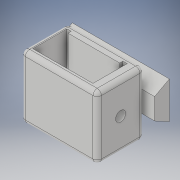
# Autodesk Inventor part: 7.2 Schienenläufer
Saved by Autodesk Inventor 2018.3 (Build 223284000, 284)
## iProperties
Created: 2018-10-11
Part Number: 7.2 Schienenläufer
Material: Generisch
Document SubType Name: Modeling
Designer: pgmadmin
Density: 1 g/cm^3
Appearance: Vorgabe
Author: pgmadmin
Autodesk Inventor part; units mm, degrees
ref_plane "YZ Plane" through (0, 0, 0) normal (1, 0, 0) x (0, 1, 0)
ref_plane "XZ Plane" through (0, 0, 0) normal (0, 1, 0) x (-1, 0, 0)
ref_plane "XY Plane" through (0, 0, 0) normal (0, 0, 1) x (1, 0, 0)
sketch "Skizze1" plane through (0, 0, 0) normal (0, 0, 1) x (1, 0, 0)
  line L0 (-14.1284, 0) -> (-14.1284, 16.2)
  line L1 (-14.1284, 16.2) -> (-12.1284, 16.2)
  line L2 (-12.1284, 16.2) -> (-12.1284, 1.6)
  line L3 (-12.1284, 1.6) -> (12.3716, 1.6)
  line L4 (12.3716, 1.6) -> (12.3716, 16.2)
  line L5 (12.3716, 16.2) -> (14.3716, 16.2)
  line L6 (14.3716, 16.2) -> (14.3716, 0)
  line L7 (14.3716, 0) -> (-14.1284, 0)
  line L8 (-16.6284, 19.2) -> (19.3716, 19.2)
  line L9 (19.3716, 19.2) -> (19.3716, -3)
  line L10 (19.3716, -3) -> (-16.6284, -3)
  line L11 (-16.6284, -3) -> (-16.6284, 19.2)
  line L12 (-12.1284, 14.7) -> (12.3716, 14.7)
  point P0 (0, 0)
  dimension "d1" = 2
  dimension "d3" = 2
  dimension "d4" = 1.6
  dimension "d5" = 3
  dimension "d7" = 2.5
  dimension "d8" = 5
  dimension "d9" = 1.5
  dimension "d26" = 3
  dimension "d27" = 28.5
  dimension "d28" = 16.2
  constraints: 26 end point, 8 perpendicular, 4 point on line, 2 parallel, 1 horizontal, 1 vertical
  measures "d1" distance of L0.end L1.end
  measures "d3" distance of L4.end L5.end
  measures "d4" distance between parallel lines of L3 L7
  measures "d5" distance between parallel lines of L10 L7
  measures "d7" distance between parallel lines of L11 L0
  measures "d8" distance between parallel lines of L9 L6
  measures "d9" distance of L1.end L12.start
  measures "d26" distance between parallel lines of L8 L1
  measures "d27" distance of L6.end L0.start
  measures "d28" distance of L0.start L0.end
extrude "Extrusion1" add sketch "Skizze1" along normal blind 30
fillet "Rundung1" radius 2 12 edges at (19.3716, 19.2, 15) (19.3716, -3, 15) (-16.6284, -3, 15) (-16.6284, 19.2, 15) (1.3716, 19.2, 30) (-16.6284, 8.1, 30) (1.3716, -3, 30) (19.3716, 8.1, 30) (19.3716, 8.1, 0) (1.3716, -3, 0) (1.3716, 19.2, 0) (-16.6284, 8.1, 0)
sketch "Skizze2" plane through (19.3716, -1, 28) normal (1, 0, 0) x (0, 0, -1)
  line L0 (0, 20.2) -> (26, 20.2) projected
  line L1 (8, 20.2) -> (4.25, 27.2)
  line L2 (4.25, 27.2) -> (21.75, 27.2)
  line L3 (21.75, 27.2) -> (18, 20.2)
  line L4 (28, 0) -> (28, 18.2) projected
  point P0 (28, 1)
  dimension "d13" = 10
  dimension "d15" = 7
  dimension "d16" = 3.75
  dimension "d17" = 3.75
  dimension "d18" = 17.5
  dimension "d19" = 10
  constraints: 6 end point, 2 point on line, 1 parallel
  measures "d13" distance of L3.end L1.start
  measures "d15" vertical distance of L1.end L1.start
  measures "d16" horizontal distance of L2.end L3.end
  measures "d17" horizontal distance of L1.start L1.end
  measures "d18" distance of L1.end L2.end
  measures "d19" distance from line of L4 L3.end
extrude "Extrusion2" add sketch "Skizze2" against normal blind 41 and the other way blind 5
sketch "Skizze5" plane through (19.3716, -1, 28) normal (1, 0, 0) x (0, 0, -1)
  circle A0 centre (13, 9.1) radius 2.4
  line L0 (13, 9.1) -> (-2, 9.1)
  line L1 (-2, 18.2) -> (-2, 0) projected
  line L2 (13, 9.1) -> (13, 20.2)
  line L3 (8, 20.2) -> (18, 20.2) projected
  line L4 (13, 9.1) -> (28, 9.1)
  point P0 (28, 1)
  dimension "d31" = 4.8
  dimension "d32" = 90
  dimension "d35" = 15
  constraints: 6 end point, 2 midpoint, 1 centre point, 1 collinear, 1 horizontal, 1 vertical
  measures "d31" diameter of A0
  measures "d32" angle of L2 L0
  measures "d35" distance between parallel lines of L1 L2
extrude "Extrusion5" cut sketch "Skizze5" against normal blind 10
